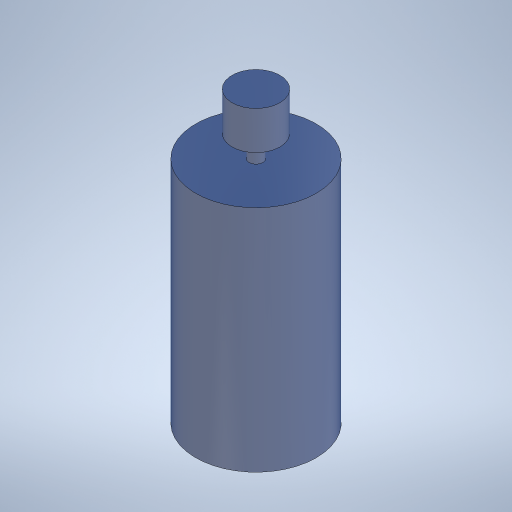
# Autodesk Inventor part: Motor
Saved by Autodesk Inventor 2023.2 (Build 272271000, 271)
## iProperties
Created: 2024-02-03
Part Number: Motor
Material: Generic
Document SubType Name: Modeling
Designer: Nathan Cai
Mass: 70 g
Surface Area: 32.9131 cm^2
Volume: 12.2674 cm^3
Density: 5.70616 g/cm^3
Appearance: Flaked Satin - Blue
Author: Nathan Cai
Autodesk Inventor part; units mm, degrees
ref_plane "YZ Plane" through (0, 0, 0) normal (1, 0, 0) x (0, 1, 0)
ref_plane "XZ Plane" through (0, 0, 0) normal (0, 1, 0) x (-1, 0, 0)
ref_plane "XY Plane" through (0, 0, 0) normal (0, 0, 1) x (1, 0, 0)
sketch "Sketch1" plane through (0, 0, 0) normal (0, 0, 1) x (1, 0, 0)
  line L0 (0, 0) -> (10, 0)
  line L1 (10, 0) -> (10, 38)
  line L2 (10, 38) -> (0, 38)
  line L3 (0, 38) -> (0, 0)
  line L4 (0, 38) -> (1.15, 38)
  line L5 (1.15, 38) -> (1.15, 48)
  line L6 (1.15, 48) -> (0, 48)
  line L7 (0, 48) -> (0, 38)
  line L8 (0, 48) -> (3.9687, 48)
  line L9 (3.9687, 48) -> (3.9688, 41.65)
  line L10 (3.9688, 41.65) -> (0, 41.65)
  line L11 (0, 41.65) -> (0, 48)
  point P0 (1.15, 41.65)
  dimension "d0" = 10
  dimension "d1" = 38
  dimension "d2" = 1.15
  dimension "d3" = 10
  dimension "d5" = 3.9688
  dimension "d6" = 6.35
  constraints: 24 end point, 6 parallel, 3 horizontal, 3 perpendicular
  measures "d0" distance of L2.end L1.end
  measures "d1" distance of L1.end L0.end
  measures "d2" distance of L6.end L5.end
  measures "d3" distance of L5.end L4.end
  measures "d5" distance of L9.end L10.end
  measures "d6" distance of L8.end L9.end
revolve "Revolution1" add sketch "Sketch1" angle 360 about axis through (0, 38, 0) along (0, -1, 0)
body "Solid1"
